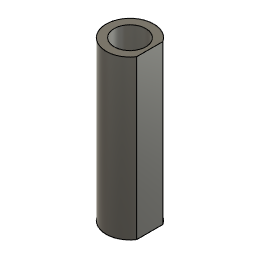
WheelBearConnector2-3 v3 (Autodesk Fusion 360 design; units mm, degrees)
Autodesk Fusion 360 part; units mm, degrees
sketch "草图1" plane through (0, 0, 0) normal (0, 1, 0) x (1, 0, 0)
  circle A0 centre (0, 0) radius 1
  line L0 (1.25, 0.8292) -> (1.25, -0.8292)
  arc A1 (1.25, 0.8292) -> (1.25, -0.8292) centre (0, 0) ccw
  dimension "d2" = 3
  dimension "d3" = 2
  constraint coincident A0.centre A1.centre
  measures "d2" diameter of A1
  measures "d3" diameter of A0
extrude "拉伸1" add sketch "草图1" along normal blind 10
sketch "草图2" plane through (0, 0, 0) normal (0, 1, 0) x (1, 0, 0)
  circle A0 centre (0, 0) radius 1
  constraint coincident A0.centre origin
extrude "拉伸2" add sketch "草图2" along normal blind 2
